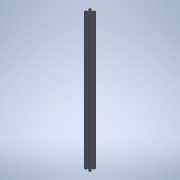
# Autodesk Inventor part: Schlitten_Profil
Saved by Autodesk Inventor 2021 (Build 250183000, 183)
## iProperties
Created: 2020-01-07
Part Number: Schlitten_Profil
Material: Aluminium
Document SubType Name: Modeling
Designer: kaebi
Density: 2.7 g/cm^3
Appearance: Eisen - Grau
Description: V-Slot Profil 20x20
Stock Number: -
Author: kaebi
Autodesk Inventor part; units mm, degrees
ref_plane "YZ Plane" through (0, 0, 0) normal (1, 0, 0) x (0, 1, 0)
ref_plane "XZ Plane" through (0, 0, 0) normal (0, 1, 0) x (-1, 0, 0)
ref_plane "XY Plane" through (0, 0, 0) normal (0, 0, 1) x (1, 0, 0)
sketch "Skizze1" plane through (0, 0, 0) normal (0, 1, 0) x (-1, 0, 0)
  line L0 (-10, 10) -> (10, 10)
  line L1 (10, 10) -> (10, -10)
  line L2 (10, -10) -> (-10, -10)
  line L3 (-10, -10) -> (-10, 10)
  line L4 (-10, 10) -> (10, -10) construction
  line L5 (10, 10) -> (-10, -10) construction
  point P0 (0, 0)
  point P1 (0, 0)
  point P2 (0, 0)
  dimension "d5" = 20
  dimension "d6" = 20
  constraints: 12 end point, 3 midpoint, 2 equal length, 1 coincident, 1 perpendicular, 1 vertical
  measures "d5" distance of L0.end L1.end
  measures "d6" distance of L1.end L2.end
extrude "Extrusion1" add sketch "Skizze1" along normal mid plane 450
sketch "Skizze2" plane through (0, 225, 0) normal (0, 1, 0) x (1, 0, 0)
  line L0 (-10, -10) -> (10, -10) projected
  line L1 (10, -10) -> (10, 10) projected
  line L2 (10, 10) -> (-10, 10) projected
  line L3 (-10, 10) -> (-10, -10) projected
  line L4 (-10, 10) -> (-10, -10) projected
  line L5 (-10, -4.5) -> (-8.5, -3)
  line L6 (-8.5, -3) -> (-8, -3)
  line L7 (-8, -3) -> (-8, -5.5)
  line L8 (-8, -5.5) -> (-6.9142, -5.5)
  line L9 (-6.9142, -5.5) -> (-4, -2.5858)
  line L10 (-4, -2.5858) -> (-4, 2.5858)
  line L11 (-4, 2.5858) -> (-6.9142, 5.5)
  line L12 (-6.9142, 5.5) -> (-8, 5.5)
  line L13 (-8, 5.5) -> (-8, 3)
  line L14 (-8, 3) -> (-8.5, 3)
  line L15 (-8.5, 3) -> (-10, 4.5)
  line L16 (-10, -4.5) -> (-10, 4.5)
  line L17 (-5.5, 6.9142) -> (-2.5858, 4)
  line L18 (-2.5858, 4) -> (2.5858, 4)
  line L19 (-5.5, 8) -> (-5.5, 6.9142)
  line L20 (-3, 8) -> (-5.5, 8)
  line L21 (-3, 8.5) -> (-3, 8)
  line L22 (2.5858, 4) -> (5.5, 6.9142)
  line L23 (3, 8) -> (3, 8.5)
  line L24 (-4.5, 10) -> (-3, 8.5)
  line L25 (5.5, 8) -> (3, 8)
  line L26 (5.5, 6.9142) -> (5.5, 8)
  line L27 (3, 8.5) -> (4.5, 10)
  line L28 (-4.5, 10) -> (4.5, 10)
  line L29 (6.9142, 5.5) -> (4, 2.5858)
  line L30 (4, 2.5858) -> (4, -2.5858)
  line L31 (8, 5.5) -> (6.9142, 5.5)
  line L32 (8, 3) -> (8, 5.5)
  line L33 (8.5, 3) -> (8, 3)
  line L34 (4, -2.5858) -> (6.9142, -5.5)
  line L35 (8, -3) -> (8.5, -3)
  line L36 (10, 4.5) -> (8.5, 3)
  line L37 (8, -5.5) -> (8, -3)
  line L38 (6.9142, -5.5) -> (8, -5.5)
  line L39 (8.5, -3) -> (10, -4.5)
  line L40 (10, 4.5) -> (10, -4.5)
  line L41 (5.5, -6.9142) -> (2.5858, -4)
  line L42 (2.5858, -4) -> (-2.5858, -4)
  line L43 (5.5, -8) -> (5.5, -6.9142)
  line L44 (3, -8) -> (5.5, -8)
  line L45 (3, -8.5) -> (3, -8)
  line L46 (-2.5858, -4) -> (-5.5, -6.9142)
  line L47 (-3, -8) -> (-3, -8.5)
  line L48 (4.5, -10) -> (3, -8.5)
  line L49 (-5.5, -8) -> (-3, -8)
  line L50 (-5.5, -6.9142) -> (-5.5, -8)
  line L51 (-3, -8.5) -> (-4.5, -10)
  line L52 (4.5, -10) -> (-4.5, -10)
  line L53 (-14, 0) -> (14, 0) projected
  circle A0 centre (0, 0) radius 2
  dimension "d9" = 360
  dimension "d13" = 8
  dimension "d14" = 2
  dimension "d15" = 2
  dimension "d16" = 9
  dimension "d17" = 6
  dimension "d18" = 11
  dimension "d19" = 4
  constraints: 96 end point, 10 point on line, 6 perpendicular, 4 equal length, 2 parallel, 1 centre point, 1 coincident, 1 collinear, 101 other
  measures "d13" distance between parallel lines of L18 L42
  measures "d14" distance between parallel lines of L46 L9
  measures "d15" distance between parallel lines of L3 L7
  measures "d16" distance of L15.end L5.start
  measures "d17" distance between parallel lines of L6 L14
  measures "d18" distance between parallel lines of L12 L8
  measures "d19" diameter of A0
extrude "Extrusion2" cut sketch "Skizze2" along normal through all both and the other way through all contours L51 L47 L49 L50 L46 L42 L41 L43 L44 L45 L48 L0 | L3 L53 L10 L9 L8 L7 L6 L5 | L3 L15 L14 L13 L12 L11 L10 L53 | L39 L35 L37 L38 L34 L30 L53 L1 | A0 L53 | L53 A0 | L53 L30 L29 L31 L32 L33 L36 L1 | L2 L27 L23 L25 L26 L22 L18 L17 L19 L20 L21 L24
